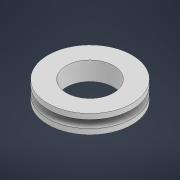
# Autodesk Inventor part: FilterPort
Saved by Autodesk Inventor 2021 (Build 250183000, 183)
## iProperties
Created: 2020-05-23
Part Number: FilterPort
Material: Generic
Document SubType Name: Modeling
Designer: Shadow
Density: 1 g/cm^3
Appearance: Default
Author: Shadow
Autodesk Inventor part; units mm, degrees
ref_plane "YZ Plane" through (0, 0, 0) normal (1, 0, 0) x (0, 1, 0)
ref_plane "XZ Plane" through (0, 0, 0) normal (0, 1, 0) x (-1, 0, 0)
ref_plane "XY Plane" through (0, 0, 0) normal (0, 0, 1) x (1, 0, 0)
sketch "Sketch1" plane through (0, 0, 0) normal (0, 1, 0) x (-1, 0, 0)
  circle A0 centre (0, 0) radius 10 construction
  circle A1 centre (0, 0) radius 16
  circle A2 centre (0, 0) radius 11
  circle A3 centre (0, 0) radius 9
  dimension "d0" = 20
  dimension "d1" = 6
  dimension "d4" = 1
  dimension "d9" = 2
  constraints: 4 centre point, 1 coincident
  measures "d0" diameter of A0
  measures "d1" radial gap between concentric circles of A0 A1
  measures "d4" radial gap between concentric circles of A0 A2
  measures "d9" radial gap between concentric circles of A2 A3
extrude "Extrusion1" add sketch "Sketch1" along normal blind 2 contours A1 | A2 | A3
extrude "Extrusion2" add sketch "Sketch1" against normal blind 3 contours A2 | A3
sketch "Sketch2" plane through (0, -3, 0) normal (0, -1, 0) x (1, 0, 0)
  circle A0 centre (0, 0) radius 16 projected
extrude "Extrusion3" add sketch "Sketch2" along normal blind 2
extrude "Extrusion4" cut sketch "Sketch1" along normal through all both and the other way through all contours A3
sketch "Sketch3" plane through (0, -5, 0) normal (0, -1, 0) x (1, 0, 0)
  circle A0 centre (0, 0) radius 11 projected
  circle A1 centre (0, 0) radius 11 projected
  circle A2 centre (0, 0) radius 10.9
  dimension "d12" = 0.1
  constraints: 1 centre point
  measures "d12" radial gap between concentric circles of A0 A2
split body "Split1" sketch "Sketch3" result two bodies curves A0 first body at (-9.377, -0.3333, 1.5239)
split body "Split2" result two bodies by plane through (0, 0, 0) normal (0, 1, 0) bodies 3 first body at (-14.0718, 0.5, -2.1538)
combine bodies "Combine1" operation type add bodies to combine 2 4
extrude "Extrusion5" cut sketch "Sketch3" against normal up to surface (2 mm away) bodies 2
move faces "Move1" translate (0, -0.1, 0) faces at (10.0739, -5, -1.5875)
equation "\"d0\" = FilterDia"
equation "\"MaskHeight\" = 125"
equation "\"FilterDia\" = 20"
equation "\"NoseWidth\" = 25"
equation "\"MaterialThickness\" = 2"
equation "\"Tol\" = 0.25"
equation "\"MaterialHardness\" = 0.3"
equation "\"ClipHeight\" = 4"
equation "\"ClipWidth\" = 5"
equation "\"ClipNeck\" = 5"
equation "\"ValveNeckDia\" = 3"
equation "\"ValveNeckLength\" = 2"
equation "\"ValveFlapDia\" = 19.25"
equation "\"LeftValve\" = 0"
equation "\"RightValve\" = 0"
equation "\"CoreScrewHeadDia\" = 9.525"
equation "\"CoreScrewLength\" = 50.8"
equation "\"CoreScrewID\" = 2.38125"
equation "\"CoreScrewOD\" = 3.96875"
equation "\"StrapAttachmentNeckDia\" = 6.5"
equation "\"StrapAttachmentNeckHeight\" = 1.5"
equation "\"StrapNoseRadialDifference\" = 2"
equation "\"StrapNoseHeight\" = 7.5"
equation "\"ZipTieThickness\" = 4"
equation "\"PinTol\" = 0.75"
equation "\"PinDia\" = 7"
equation "\"PinDepth\" = 5"
body "Solid2"
body "Solid5"
